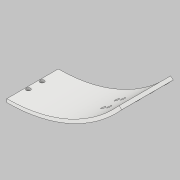
# Autodesk Inventor part: CW003
Saved by Autodesk Inventor 2017 (Build 210142000, 142)
## iProperties
Created: 2017-05-23
Part Number: CW003
Material: ABS Plastic
Document SubType Name: Modeling
Designer: zallen
Density: 1.06 g/cm^3
Appearance: CR White
Author: zallen
Autodesk Inventor part; units mm, degrees
ref_plane "YZ Plane" through (0, 0, 0) normal (1, 0, 0) x (0, 1, 0)
sketch "Sketch1" plane through (0, 0, 0) normal (0, 0, 1) x (1, 0, 0)
  circle A0 centre (0, 225) radius 225 construction
  circle A1 centre (0, 225) radius 220 construction
  line L0 (0, 0) -> (0, 5)
  arc A2 (0, 0) -> (167.5, 74.771) centre (0, 225) ccw
  line L1 (167.5, 74.771) -> (163.7778, 78.1094)
  arc A3 (0, 5) -> (163.7778, 78.1094) centre (0, 225) ccw
  dimension "d0" = 450
  dimension "d1" = 5
  dimension "d2" = 5
  dimension "d6" = 167.5
  constraints: 8 point on circle, 4 centre point, 4 concentric, 4 end point, 1 vertical, 1 vertical alignment
  measures "d0" diameter of A0
  measures "d1" radial gap between concentric circles of A0 A1
  measures "d2" distance of L1.start L1.end
  measures "d6" horizontal distance of L1.start L0.start
extrude "Extrusion1" add sketch "Sketch1" along normal blind 75
ref_plane "Work Plane2" through (0, 0, 0) normal (0, -1, 0) x (1, 0, 0)
sketch "Sketch3" plane through (0, 0, 0) normal (0, -1, 0) x (1, 0, 0)
  circle A0 centre (4, 47.5) radius 3
  circle A1 centre (4, 27.5) radius 3
  point P0 (0, 0)
  dimension "d15" = 6
  dimension "d16" = 6
  dimension "d17" = 27.5
  dimension "d18" = 20
  dimension "d19" = 4
  constraints: 2 centre point, 1 vertical alignment
  measures "d15" diameter of A0
  measures "d16" diameter of A1
  measures "d17" vertical distance of point (0, 0) A1.centre
  measures "d18" distance of A1.centre A0.centre
  measures "d19" horizontal distance of A1.centre point (0, 0)
extrude "Extrusion3" cut sketch "Sketch3" along normal through all both and the other way through all
ref_plane "Work Plane3" through (167.5, 74.771, 0) normal (0.7444, -0.6677, 0) x (0.6677, 0.7444, 0)
sketch "Sketch4" plane through (167.5, 74.771, 0) normal (0.7444, -0.6677, 0) x (0.6677, 0.7444, 0)
  circle A0 centre (-55, 47.5) radius 3
  circle A1 centre (-55, 27.5) radius 3
  line L0 (-167.5, 0) -> (0, 0) projected
  line L1 (0, 0) -> (0, 75) projected
  circle A2 centre (-5, 47.5) radius 3
  circle A3 centre (-5, 27.5) radius 3
  circle A4 centre (-65, 27.5) radius 3
  circle A5 centre (-65, 47.5) radius 3
  dimension "d22" = 6
  dimension "d23" = 6
  dimension "d24" = 27.5
  dimension "d25" = 20
  dimension "d26" = 55
  dimension "d29" = 6
  dimension "d30" = 6
  dimension "d31" = 5
  dimension "d32" = 6
  dimension "d33" = 6
  dimension "d34" = 10
  constraints: 6 centre point, 4 horizontal alignment, 3 vertical alignment
  measures "d22" diameter of A0
  measures "d23" diameter of A1
  measures "d24" distance from line of L0 A1.centre
  measures "d25" distance of A1.centre A0.centre
  measures "d26" distance from line of L1 A1.centre
  measures "d29" diameter of A2
  measures "d30" diameter of A3
  measures "d31" horizontal distance of A3.centre L0.end
  measures "d32" diameter of A4
  measures "d33" diameter of A5
  measures "d34" distance of A4.centre A1.centre
extrude "Extrusion4" cut sketch "Sketch4" along normal through all both and the other way through all
body "Solid1"
